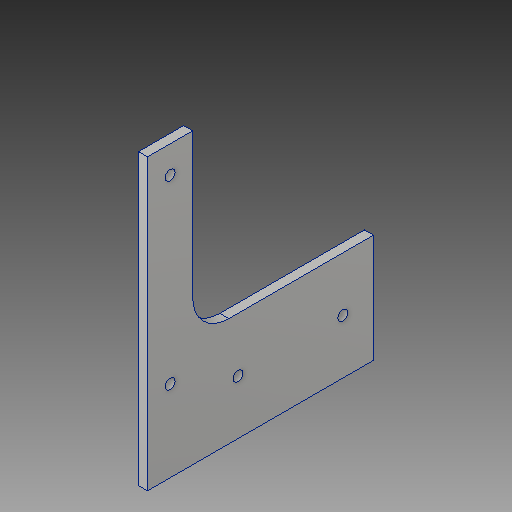
# Autodesk Inventor part: Front Brace 2
Saved by Autodesk Inventor 2019.4 (Build 234330000, 330)
## iProperties
Created: 2020-01-06
Part Number: Front Brace 2
Material: Aluminum 6061
Document SubType Name: Modeling
Designer: Mark
Mass: 134.876 g
Surface Area: 231.343 cm^2
Volume: 49.954 cm^3
Density: 2.7 g/cm^3
Appearance: Aluminum - Flat
Author: Mark
Autodesk Inventor part; units mm, degrees
ref_plane "YZ Plane" through (0, 0, 0) normal (1, 0, 0) x (0, 1, 0)
ref_plane "XZ Plane" through (0, 0, 0) normal (0, 1, 0) x (-1, 0, 0)
ref_plane "XY Plane" through (0, 0, 0) normal (0, 0, 1) x (1, 0, 0)
sketch "Sketch1" plane through (0, 0, 0) normal (1, 0, 0) x (0, 1, 0)
  line L0 (0, 0) -> (160, 0)
  line L1 (160, 0) -> (160, -25)
  line L2 (160, -25) -> (0, -25)
  line L3 (0, -25) -> (0, 0)
  line L4 (0, -25) -> (60, -25)
  line L5 (60, -25) -> (60, -125)
  line L6 (60, -125) -> (0, -125)
  line L7 (0, -125) -> (0, -25)
  dimension "d0" = 160
  dimension "d1" = 25
  dimension "d2" = 60
  dimension "d3" = 100
  constraints: 16 end point, 4 parallel, 2 horizontal, 2 perpendicular
  measures "d0" distance of L1.end L2.end
  measures "d1" distance of L0.end L1.end
  measures "d2" distance of L5.end L6.end
  measures "d3" distance of L4.end L5.end
extrude "Extrusion1" add sketch "Sketch1" along normal blind 5
fillet "Fillet1" radius 20 1 edges at (2.5, 60, -25)
sketch "Sketch2" plane through (0, 0, 0) normal (-1, 0, 0) x (0, 0, 1)
  circle A0 centre (-12.5, 45) radius 2.75
  circle A1 centre (-12.5, 145) radius 2.75
  line L0 (-125, 0) -> (0, 0) projected
  line L1 (0, 0) -> (0, 160) projected
  circle A2 centre (-50, 30) radius 2.75
  circle A3 centre (-108, 30) radius 2.75
  dimension "d7" = 5.5
  dimension "d8" = 5.5
  dimension "d9" = 100
  dimension "d10" = 45
  dimension "d11" = 12.5
  dimension "d12" = 12.5
  dimension "d15" = 5.5
  dimension "d16" = 5.5
  dimension "d17" = 50
  dimension "d18" = 58
  dimension "d19" = 30
  dimension "d20" = 30
  constraints: 4 centre point
  measures "d7" diameter of A0
  measures "d8" diameter of A1
  measures "d9" distance of A0.centre A1.centre
  measures "d10" distance from line of L0 A0.centre
  measures "d11" distance from line of L1 A0.centre
  measures "d12" distance from line of L1 A1.centre
  measures "d15" diameter of A2
  measures "d16" diameter of A3
  measures "d17" distance from line of L1 A2.centre
  measures "d18" distance of A3.centre A2.centre
  measures "d19" distance from line of L0 A3.centre
  measures "d20" distance from line of L0 A2.centre
extrude "Extrusion2" cut sketch "Sketch2" against normal blind 5
body "Solid1"
